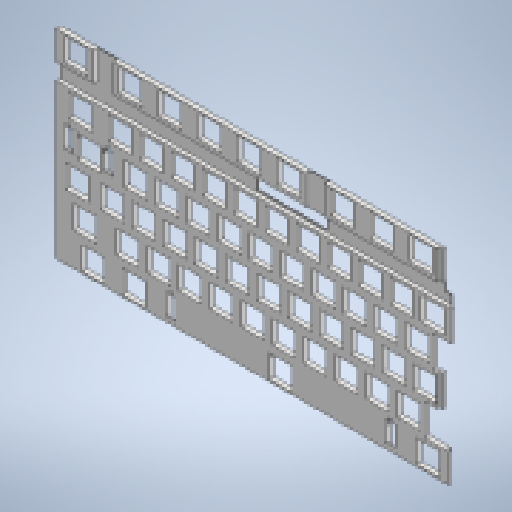
# Autodesk Inventor part: Left Plate
Saved by Autodesk Inventor 2025 (Build 290162000, 162)
## iProperties
Created: 2024-08-15
Part Number: Left Plate
Material: Generic
Document SubType Name: Modeling
Designer: adam
Density: 1 g/cm^3
Appearance: Default
Author: adam
Autodesk Inventor part; units mm, degrees
(part 1 of 2)
ref_plane "YZ Plane" through (0, 0, 0) normal (1, 0, 0) x (0, 1, 0)
ref_plane "XZ Plane" through (0, 0, 0) normal (0, 1, 0) x (-1, 0, 0)
ref_plane "XY Plane" through (0, 0, 0) normal (0, 0, 1) x (1, 0, 0)
sketch "Sketch1" plane through (0, 0, 0) normal (0, 0, 1) x (1, 0, 0)
  line L0 (356, -163) -> (40, -163) construction
  line L1 (356, -42) -> (356, -163) construction
  line L2 (40, -42) -> (356, -42) construction
  line L3 (40, -163) -> (40, -42) construction
  circle A0 centre (58.6, -159.6) radius 0.725 construction
  circle A1 centre (63, -154.9) radius 2.55 construction
  circle A2 centre (65.6, -160.65) radius 0.725 construction
  circle A3 centre (83.1, -159.6) radius 0.725 construction
  circle A4 centre (90.1, -160.65) radius 0.725 construction
  circle A5 centre (87.5, -154.9) radius 2.55 construction
  line L4 (107.125, -161.9) -> (113.125, -161.9) construction
  line L5 (107.125, -145.9) -> (107.125, -161.9) construction
  line L6 (113.125, -145.9) -> (107.125, -145.9) construction
  line L7 (113.125, -161.9) -> (113.125, -145.9) construction
  circle A6 centre (53.1, -140.5) radius 0.725 construction
  circle A7 centre (60.1, -141.55) radius 0.725 construction
  circle A8 centre (79.35, -140.5) radius 0.725 construction
  circle A9 centre (57.5, -135.8) radius 2.55 construction
  circle A10 centre (86.35, -141.55) radius 0.725 construction
  circle A11 centre (98.35, -140.5) radius 0.725 construction
  circle A12 centre (105.35, -141.55) radius 0.725 construction
  circle A13 centre (117.35, -140.5) radius 0.725 construction
  circle A14 centre (83.75, -135.8) radius 2.55 construction
  circle A15 centre (102.75, -135.8) radius 2.55 construction
  circle A16 centre (121.75, -135.8) radius 2.55 construction
  circle A17 centre (179.475, -160.65) radius 0.725 construction
  circle A18 centre (172.475, -159.6) radius 0.725 construction
  circle A19 centre (176.875, -154.9) radius 2.55 construction
  circle A20 centre (124.35, -141.55) radius 0.725 construction
  circle A21 centre (136.35, -140.5) radius 0.725 construction
  circle A22 centre (143.35, -141.55) radius 0.725 construction
  circle A23 centre (155.35, -140.5) radius 0.725 construction
  circle A24 centre (140.75, -135.8) radius 2.55 construction
  circle A25 centre (159.75, -135.8) radius 2.55 construction
  circle A26 centre (162.35, -141.55) radius 0.725 construction
  circle A27 centre (174.35, -140.5) radius 0.725 construction
  circle A28 centre (181.35, -141.55) radius 0.725 construction
  circle A29 centre (193.35, -140.5) radius 0.725 construction
  circle A30 centre (178.75, -135.8) radius 2.55 construction
  circle A31 centre (197.75, -135.8) radius 2.55 construction
  circle A32 centre (48.6, -121.4) radius 0.725 construction
  circle A33 centre (55.6, -122.45) radius 0.725 construction
  circle A34 centre (70.1, -121.4) radius 0.725 construction
  circle A35 centre (77.1, -122.45) radius 0.725 construction
  circle A36 centre (89.1, -121.4) radius 0.725 construction
  circle A37 centre (96.1, -122.45) radius 0.725 construction
  circle A38 centre (108.1, -121.4) radius 0.725 construction
  circle A39 centre (115.1, -122.45) radius 0.725 construction
  circle A40 centre (53, -116.7) radius 2.55 construction
  circle A41 centre (74.5, -116.7) radius 2.55 construction
  circle A42 centre (93.5, -116.7) radius 2.55 construction
  circle A43 centre (112.5, -116.7) radius 2.55 construction
  circle A44 centre (127.1, -121.4) radius 0.725 construction
  circle A45 centre (134.1, -122.45) radius 0.725 construction
  circle A46 centre (146.1, -121.4) radius 0.725 construction
  circle A47 centre (153.1, -122.45) radius 0.725 construction
  circle A48 centre (165.1, -121.4) radius 0.725 construction
  circle A49 centre (172.1, -122.45) radius 0.725 construction
  circle A50 centre (184.1, -121.4) radius 0.725 construction
  circle A51 centre (191.1, -122.45) radius 0.725 construction
  circle A52 centre (131.5, -116.7) radius 2.55 construction
  circle A53 centre (150.5, -116.7) radius 2.55 construction
  circle A54 centre (169.5, -116.7) radius 2.55 construction
  circle A55 centre (188.5, -116.7) radius 2.55 construction
  circle A56 centre (261.85, -159.6) radius 0.725 construction
  circle A57 centre (268.85, -160.65) radius 0.725 construction
  circle A58 centre (266.25, -154.9) radius 2.55 construction
  line L8 (240.625, -161.9) -> (246.625, -161.9) construction
  line L9 (240.625, -145.9) -> (240.625, -161.9) construction
  line L10 (246.625, -145.9) -> (240.625, -145.9) construction
  line L11 (246.625, -161.9) -> (246.625, -145.9) construction
  circle A59 centre (200.35, -141.55) radius 0.725 construction
  circle A60 centre (212.35, -140.5) radius 0.725 construction
  circle A61 centre (219.35, -141.55) radius 0.725 construction
  circle A62 centre (231.35, -140.5) radius 0.725 construction
  circle A63 centre (216.75, -135.8) radius 2.55 construction
  circle A64 centre (235.75, -135.8) radius 2.55 construction
  circle A65 centre (238.35, -141.55) radius 0.725 construction
  circle A66 centre (250.35, -140.5) radius 0.725 construction
  circle A67 centre (257.35, -141.55) radius 0.725 construction
  circle A68 centre (269.35, -140.5) radius 0.725 construction
  circle A69 centre (276.35, -141.55) radius 0.725 construction
  circle A70 centre (254.75, -135.8) radius 2.55 construction
  circle A71 centre (273.75, -135.8) radius 2.55 construction
  circle A72 centre (283.85, -159.6) radius 0.725 construction
  circle A73 centre (290.85, -160.65) radius 0.725 construction
  circle A74 centre (288.25, -154.9) radius 2.55 construction
  circle A75 centre (302.85, -159.6) radius 0.725 construction
  circle A76 centre (309.85, -160.65) radius 0.725 construction
  circle A77 centre (307.25, -154.9) radius 2.55 construction
  circle A78 centre (321.85, -159.6) radius 0.725 construction
  circle A79 centre (328.85, -160.65) radius 0.725 construction
  circle A80 centre (326.25, -154.9) radius 2.55 construction
  circle A81 centre (340.85, -159.6) radius 0.725 construction
  circle A82 centre (347.85, -160.65) radius 0.725 construction
  circle A83 centre (345.25, -154.9) radius 2.55 construction
  circle A84 centre (295.6, -140.5) radius 0.725 construction
  circle A85 centre (302.6, -141.55) radius 0.725 construction
  circle A86 centre (300, -135.8) radius 2.55 construction
  circle A87 centre (321.85, -140.5) radius 0.725 construction
  circle A88 centre (328.85, -141.55) radius 0.725 construction
  circle A89 centre (353.5, -141.62) radius 0.5 construction
  circle A90 centre (326.25, -135.8) radius 2.55 construction
  circle A91 centre (353.5, -139.08) radius 0.5 construction
  circle A92 centre (353.5, -136.54) radius 0.5 construction
  circle A93 centre (353.5, -134) radius 0.5 construction
  circle A94 centre (203.1, -121.4) radius 0.725 construction
  circle A95 centre (210.1, -122.45) radius 0.725 construction
  circle A96 centre (222.1, -121.4) radius 0.725 construction
  circle A97 centre (229.1, -122.45) radius 0.725 construction
  circle A98 centre (241.1, -121.4) radius 0.725 construction
  circle A99 centre (248.1, -122.45) radius 0.725 construction
  circle A100 centre (260.1, -121.4) radius 0.725 construction
  circle A101 centre (267.1, -122.45) radius 0.725 construction
  circle A102 centre (207.5, -116.7) radius 2.55 construction
  circle A103 centre (226.5, -116.7) radius 2.55 construction
  circle A104 centre (245.5, -116.7) radius 2.55 construction
  circle A105 centre (264.5, -116.7) radius 2.55 construction
  circle A106 centre (279.1, -121.4) radius 0.725 construction
  circle A107 centre (286.1, -122.45) radius 0.725 construction
  circle A108 centre (298.1, -121.4) radius 0.725 construction
  circle A109 centre (305.1, -122.45) radius 0.725 construction
  line L12 (315, -122.25) -> (330, -122.25) construction
  line L13 (315, -116.25) -> (315, -122.25) construction
  line L14 (330, -116.25) -> (315, -116.25) construction
  line L15 (330, -122.25) -> (330, -116.25) construction
  circle A110 centre (283.5, -116.7) radius 2.55 construction
  circle A111 centre (302.5, -116.7) radius 2.55 construction
  circle A112 centre (328.675, -111.675) radius 0.725 construction
  circle A113 centre (323.975, -107.275) radius 2.55 construction
  circle A114 centre (329.725, -104.675) radius 0.725 construction
  circle A115 centre (62.6, -103.35) radius 0.725 construction
  circle A116 centre (55.6, -102.3) radius 0.725 construction
  circle A117 centre (60, -97.6) radius 2.55 construction
  line L16 (45, -103.6) -> (51, -103.6) construction
  line L17 (45, -88.6) -> (45, -103.6) construction
  line L18 (51, -88.6) -> (45, -88.6) construction
  line L19 (51, -103.6) -> (51, -88.6) construction
  line L20 (69, -103.6) -> (75, -103.6) construction
  line L21 (69, -88.6) -> (69, -103.6) construction
  line L22 (75, -88.6) -> (69, -88.6) construction
  line L23 (75, -103.6) -> (75, -88.6) construction
  circle A118 centre (91.35, -103.35) radius 0.725 construction
  circle A119 centre (84.35, -102.3) radius 0.725 construction
  circle A120 centre (88.75, -97.6) radius 2.55 construction
  circle A121 centre (110.35, -103.35) radius 0.725 construction
  circle A122 centre (103.35, -102.3) radius 0.725 construction
  circle A123 centre (107.75, -97.6) radius 2.55 construction
  circle A124 centre (57.6, -84.25) radius 0.725 construction
  circle A125 centre (81.6, -84.25) radius 0.725 construction
  circle A126 centre (50.6, -83.2) radius 0.725 construction
  circle A127 centre (55, -78.5) radius 2.55 construction
  circle A128 centre (74.6, -83.2) radius 0.725 construction
  circle A129 centre (79, -78.5) radius 2.55 construction
  circle A130 centre (100.6, -84.25) radius 0.725 construction
  circle A131 centre (119.6, -84.25) radius 0.725 construction
  circle A132 centre (93.6, -83.2) radius 0.725 construction
  circle A133 centre (98, -78.5) radius 2.55 construction
  circle A134 centre (112.6, -83.2) radius 0.725 construction
  circle A135 centre (117, -78.5) radius 2.55 construction
  circle A136 centre (129.35, -103.35) radius 0.725 construction
  circle A137 centre (122.35, -102.3) radius 0.725 construction
  circle A138 centre (141.35, -102.3) radius 0.725 construction
  circle A139 centre (126.75, -97.6) radius 2.55 construction
  circle A140 centre (148.35, -103.35) radius 0.725 construction
  circle A141 centre (160.35, -102.3) radius 0.725 construction
  circle A142 centre (145.75, -97.6) radius 2.55 construction
  circle A143 centre (167.35, -103.35) radius 0.725 construction
  circle A144 centre (179.35, -102.3) radius 0.725 construction
  circle A145 centre (164.75, -97.6) radius 2.55 construction
  circle A146 centre (186.35, -103.35) radius 0.725 construction
  circle A147 centre (198.35, -102.3) radius 0.725 construction
  circle A148 centre (183.75, -97.6) radius 2.55 construction
  circle A149 centre (138.6, -84.25) radius 0.725 construction
  circle A150 centre (157.6, -84.25) radius 0.725 construction
  circle A151 centre (131.6, -83.2) radius 0.725 construction
  circle A152 centre (136, -78.5) radius 2.55 construction
  circle A153 centre (150.6, -83.2) radius 0.725 construction
  circle A154 centre (155, -78.5) radius 2.55 construction
  circle A155 centre (176.6, -84.25) radius 0.725 construction
  circle A156 centre (195.6, -84.25) radius 0.725 construction
  circle A157 centre (169.6, -83.2) radius 0.725 construction
  circle A158 centre (174, -78.5) radius 2.55 construction
  circle A159 centre (188.6, -83.2) radius 0.725 construction
  circle A160 centre (193, -78.5) radius 2.55 construction
  circle A161 centre (48.1, -54.7) radius 0.725 construction
  circle A162 centre (55.1, -55.75) radius 0.725 construction
  circle A163 centre (81.1, -54.7) radius 0.725 construction
  circle A164 centre (52.5, -50) radius 2.55 construction
  circle A165 centre (88.1, -55.75) radius 0.725 construction
  circle A166 centre (105.1, -54.7) radius 0.725 construction
  circle A167 centre (112.1, -55.75) radius 0.725 construction
  circle A168 centre (85.5, -50) radius 2.55 construction
  circle A169 centre (109.5, -50) radius 2.55 construction
  circle A170 centre (163.5, -66.25) radius 0.425 construction
  circle A171 centre (166, -66.25) radius 0.425 construction
  circle A172 centre (168.5, -66.25) radius 0.425 construction
  circle A173 centre (171, -66.25) radius 0.425 construction
  circle A174 centre (173.5, -66.25) radius 0.425 construction
  circle A175 centre (176, -66.25) radius 0.425 construction
  circle A176 centre (178.5, -66.25) radius 0.425 construction
  circle A177 centre (162.25, -63.75) radius 0.425 construction
  circle A178 centre (164.75, -63.75) radius 0.425 construction
  circle A179 centre (167.25, -63.75) radius 0.425 construction
  circle A180 centre (169.75, -63.75) radius 0.425 construction
  circle A181 centre (172.25, -63.75) radius 0.425 construction
  circle A182 centre (174.75, -63.75) radius 0.425 construction
  circle A183 centre (177.25, -63.75) radius 0.425 construction
  circle A184 centre (179.75, -63.75) radius 0.425 construction
  circle A185 centre (181, -66.25) radius 0.425 construction
  circle A186 centre (183.5, -66.25) radius 0.425 construction
  circle A187 centre (186, -66.25) radius 0.425 construction
  circle A188 centre (188.5, -66.25) radius 0.425 construction
  circle A189 centre (191, -66.25) radius 0.425 construction
  circle A190 centre (193.5, -66.25) radius 0.425 construction
  circle A191 centre (196, -66.25) radius 0.425 construction
  circle A192 centre (198.5, -66.25) radius 0.425 construction
  circle A193 centre (182.25, -63.75) radius 0.425 construction
  circle A194 centre (184.75, -63.75) radius 0.425 construction
  circle A195 centre (187.25, -63.75) radius 0.425 construction
  circle A196 centre (189.75, -63.75) radius 0.425 construction
  circle A197 centre (192.25, -63.75) radius 0.425 construction
  circle A198 centre (194.75, -63.75) radius 0.425 construction
  circle A199 centre (197.25, -63.75) radius 0.425 construction
  circle A200 centre (129.1, -54.7) radius 0.725 construction
  circle A201 centre (136.1, -55.75) radius 0.725 construction
  circle A202 centre (153.1, -54.7) radius 0.725 construction
  circle A203 centre (160.1, -55.75) radius 0.725 construction
  circle A204 centre (133.5, -50) radius 2.55 construction
  circle A205 centre (157.5, -50) radius 2.55 construction
  circle A206 centre (177.1, -54.7) radius 0.725 construction
  circle A207 centre (184.1, -55.75) radius 0.725 construction
  circle A208 centre (181.5, -50) radius 2.55 construction
  circle A209 centre (205.35, -103.35) radius 0.725 construction
  circle A210 centre (217.35, -102.3) radius 0.725 construction
  circle A211 centre (202.75, -97.6) radius 2.55 construction
  circle A212 centre (224.35, -103.35) radius 0.725 construction
  circle A213 centre (236.35, -102.3) radius 0.725 construction
  circle A214 centre (221.75, -97.6) radius 2.55 construction
  circle A215 centre (243.35, -103.35) radius 0.725 construction
  circle A216 centre (255.35, -102.3) radius 0.725 construction
  circle A217 centre (240.75, -97.6) radius 2.55 construction
  circle A218 centre (262.35, -103.35) radius 0.725 construction
  circle A219 centre (274.35, -102.3) radius 0.725 construction
  circle A220 centre (259.75, -97.6) radius 2.55 construction
  circle A221 centre (214.6, -84.25) radius 0.725 construction
  circle A222 centre (233.6, -84.25) radius 0.725 construction
  circle A223 centre (207.6, -83.2) radius 0.725 construction
  circle A224 centre (212, -78.5) radius 2.55 construction
  circle A225 centre (226.6, -83.2) radius 0.725 construction
  circle A226 centre (231, -78.5) radius 2.55 construction
  circle A227 centre (252.6, -84.25) radius 0.725 construction
  circle A228 centre (271.6, -84.25) radius 0.725 construction
  circle A229 centre (245.6, -83.2) radius 0.725 construction
  circle A230 centre (250, -78.5) radius 2.55 construction
  circle A231 centre (264.6, -83.2) radius 0.725 construction
  circle A232 centre (269, -78.5) radius 2.55 construction
  circle A233 centre (281.35, -103.35) radius 0.725 construction
  circle A234 centre (293.35, -102.3) radius 0.725 construction
  circle A235 centre (278.75, -97.6) radius 2.55 construction
  circle A236 centre (300.35, -103.35) radius 0.725 construction
  circle A237 centre (297.75, -97.6) radius 2.55 construction
  line L24 (315, -98.25) -> (330, -98.25) construction
  line L25 (315, -92.25) -> (315, -98.25) construction
  line L26 (330, -92.25) -> (315, -92.25) construction
  line L27 (330, -98.25) -> (330, -92.25) construction
  circle A238 centre (290.6, -84.25) radius 0.725 construction
  circle A239 centre (309.6, -84.25) radius 0.725 construction
  circle A240 centre (283.6, -83.2) radius 0.725 construction
  circle A241 centre (288, -78.5) radius 2.55 construction
  circle A242 centre (302.6, -83.2) radius 0.725 construction
  circle A243 centre (307, -78.5) radius 2.55 construction
  circle A244 centre (328.6, -84.25) radius 0.725 construction
  circle A245 centre (347.6, -84.25) radius 0.725 construction
  circle A246 centre (321.6, -83.2) radius 0.725 construction
  circle A247 centre (326, -78.5) radius 2.55 construction
  circle A248 centre (340.6, -83.2) radius 0.725 construction
  circle A249 centre (345, -78.5) radius 2.55 construction
  circle A250 centre (201, -66.25) radius 0.425 construction
  circle A251 centre (199.75, -63.75) radius 0.425 construction
  circle A252 centre (259, -74) radius 1.6 construction
  circle A253 centre (209.6, -54.7) radius 0.725 construction
  circle A254 centre (216.6, -55.75) radius 0.725 construction
  circle A255 centre (233.6, -54.7) radius 0.725 construction
  circle A256 centre (214, -50) radius 2.55 construction
  circle A257 centre (238, -50) radius 2.55 construction
  circle A258 centre (240.6, -55.75) radius 0.725 construction
  circle A259 centre (257.6, -54.7) radius 0.725 construction
  circle A260 centre (264.6, -55.75) radius 0.725 construction
  circle A261 centre (262, -50) radius 2.55 construction
  circle A262 centre (281.6, -54.7) radius 0.725 construction
  circle A263 centre (288.6, -55.75) radius 0.725 construction
  circle A264 centre (305.6, -54.7) radius 0.725 construction
  circle A265 centre (312.6, -55.75) radius 0.725 construction
  circle A266 centre (286, -50) radius 2.55 construction
  circle A267 centre (310, -50) radius 2.55 construction
  circle A268 centre (339.1, -54.7) radius 0.725 construction
  circle A269 centre (346.1, -55.75) radius 0.725 construction
  circle A270 centre (343.5, -50) radius 2.55 construction
  line L28 (277.25, -163) -> (277.25, -145.35) construction
  line L29 (277.25, -145.35) -> (264.25, -145.35) construction
  line L30 (264.25, -145.35) -> (264.25, -126.25) construction
  line L31 (264.25, -126.25) -> (274, -126.25) construction
  line L32 (274, -126.25) -> (274, -107.15) construction
  line L33 (274, -107.15) -> (269.25, -107.15) construction
  line L34 (269.25, -107.15) -> (269.25, -88.05) construction
  line L35 (269.25, -88.05) -> (278.5, -88.05) construction
  line L36 (278.5, -88.05) -> (278.5, -64.25) construction
  line L37 (274, -42) -> (274, -64.25) construction
  line L38 (274, -64.25) -> (278.5, -64.25) construction
  line L39 (262, -50) -> (274, -50) construction
  line L40 (274, -50) -> (286, -50) construction
  line L41 (269, -78.5) -> (278.5, -78.5) construction
  line L42 (278.5, -78.5) -> (288, -78.5) construction
  line L43 (259.75, -97.6) -> (269.25, -97.6) construction
  line L44 (269.25, -97.6) -> (278.75, -97.6) construction
  line L45 (264.5, -116.7) -> (274, -116.7) construction
  line L46 (283.5, -116.7) -> (274, -116.7) construction
  line L47 (254.75, -135.8) -> (264.25, -135.8) construction
  line L48 (273.75, -135.8) -> (264.25, -135.8) construction
  line L49 (266.25, -154.9) -> (277.25, -154.9) construction
  line L50 (288.25, -154.9) -> (277.25, -154.9) construction
  line L51 (273.75, -135.8) -> (273.75, -145.35) construction
  line L52 (273.75, -145.35) -> (273.75, -154.9) construction
  line L53 (269.35, -140.5) -> (269.35, -135.8) construction
  line L54 (269.35, -135.8) -> (269.35, -126.25) construction
  line L55 (269.35, -126.25) -> (269.35, -116.7) construction
  line L56 (271.75, -116.7) -> (271.75, -107.15) construction
  line L57 (271.75, -107.15) -> (271.75, -97.6) construction
  line L58 (271.75, -97.6) -> (271.75, -88.05) construction
  line L59 (271.75, -88.05) -> (271.75, -78.5) construction
  line L60 (276.25, -78.5) -> (276.25, -64.25) construction
  line L61 (276.25, -64.25) -> (276.25, -50) construction
  line L62 (273.9, -126.15) -> (264.15, -126.15)
  line L63 (264.15, -126.15) -> (264.15, -145.45)
  line L64 (264.15, -145.45) -> (277.15, -145.45)
  line L65 (277.15, -145.45) -> (277.15, -163)
  line L66 (277.15, -163) -> (40, -163)
  line L67 (40, -163) -> (40, -42)
  line L68 (40, -42) -> (273.9, -42)
  line L69 (273.9, -126.15) -> (273.9, -107.25)
  line L70 (273.9, -107.25) -> (269.15, -107.25)
  line L71 (269.15, -107.25) -> (269.15, -87.95)
  line L72 (269.15, -87.95) -> (278.4, -87.95)
  line L73 (278.4, -87.95) -> (278.4, -64.35)
  line L74 (278.4, -64.35) -> (273.9, -64.35)
  line L75 (273.9, -64.35) -> (273.9, -42)
  line L76 (45.4975, -42.9975) -> (59.5025, -42.9975)
  line L77 (59.5025, -42.9975) -> (59.5025, -57.0025)
  line L78 (59.5025, -57.0025) -> (45.4975, -57.0025)
  line L79 (45.4975, -57.0025) -> (45.4975, -42.9975)
  line L80 (45.4975, -42.9975) -> (59.5025, -57.0025) construction
  line L81 (59.5025, -42.9975) -> (45.4975, -57.0025) construction
  line L82 (78.4975, -42.9975) -> (92.5025, -42.9975)
  line L83 (92.5025, -42.9975) -> (92.5025, -57.0025)
  line L84 (92.5025, -57.0025) -> (78.4975, -57.0025)
  line L85 (78.4975, -57.0025) -> (78.4975, -42.9975)
  line L86 (78.4975, -42.9975) -> (92.5025, -57.0025) construction
  line L87 (92.5025, -42.9975) -> (78.4975, -57.0025) construction
  line L88 (102.4975, -42.9975) -> (116.5025, -42.9975)
  line L89 (116.5025, -42.9975) -> (116.5025, -57.0025)
  line L90 (116.5025, -57.0025) -> (102.4975, -57.0025)
  line L91 (102.4975, -57.0025) -> (102.4975, -42.9975)
  line L92 (102.4975, -42.9975) -> (116.5025, -57.0025) construction
  line L93 (116.5025, -42.9975) -> (102.4975, -57.0025) construction
  line L94 (126.4975, -42.9975) -> (140.5025, -42.9975)
  line L95 (140.5025, -42.9975) -> (140.5025, -57.0025)
  line L96 (140.5025, -57.0025) -> (126.4975, -57.0025)
  line L97 (126.4975, -57.0025) -> (126.4975, -42.9975)
  line L98 (126.4975, -42.9975) -> (140.5025, -57.0025) construction
  line L99 (140.5025, -42.9975) -> (126.4975, -57.0025) construction
  line L100 (150.4975, -42.9975) -> (164.5025, -42.9975)
  line L101 (164.5025, -42.9975) -> (164.5025, -57.0025)
  line L102 (164.5025, -57.0025) -> (150.4975, -57.0025)
  line L103 (150.4975, -57.0025) -> (150.4975, -42.9975)
  line L104 (150.4975, -42.9975) -> (164.5025, -57.0025) construction
  line L105 (164.5025, -42.9975) -> (150.4975, -57.0025) construction
  line L106 (174.4975, -42.9975) -> (188.5025, -42.9975)
  line L107 (188.5025, -42.9975) -> (188.5025, -57.0025)
  line L108 (188.5025, -57.0025) -> (174.4975, -57.0025)
  line L109 (174.4975, -57.0025) -> (174.4975, -42.9975)
  line L110 (174.4975, -42.9975) -> (188.5025, -57.0025) construction
  line L111 (188.5025, -42.9975) -> (174.4975, -57.0025) construction
  line L112 (206.9975, -42.9975) -> (221.0025, -42.9975)
  line L113 (221.0025, -42.9975) -> (221.0025, -57.0025)
  line L114 (221.0025, -57.0025) -> (206.9975, -57.0025)
  line L115 (206.9975, -57.0025) -> (206.9975, -42.9975)
  line L116 (206.9975, -42.9975) -> (221.0025, -57.0025) construction
  line L117 (221.0025, -42.9975) -> (206.9975, -57.0025) construction
  line L118 (230.9975, -42.9975) -> (245.0025, -42.9975)
  line L119 (245.0025, -42.9975) -> (245.0025, -57.0025)
  line L120 (245.0025, -57.0025) -> (230.9975, -57.0025)
  line L121 (230.9975, -57.0025) -> (230.9975, -42.9975)
  line L122 (230.9975, -42.9975) -> (245.0025, -57.0025) construction
  line L123 (245.0025, -42.9975) -> (230.9975, -57.0025) construction
  line L124 (254.9975, -42.9975) -> (269.0025, -42.9975)
  line L125 (269.0025, -42.9975) -> (269.0025, -57.0025)
  line L126 (269.0025, -57.0025) -> (254.9975, -57.0025)
  line L127 (254.9975, -57.0025) -> (254.9975, -42.9975)
  line L128 (254.9975, -42.9975) -> (269.0025, -57.0025) construction
  line L129 (269.0025, -42.9975) -> (254.9975, -57.0025) construction
  line L130 (47.9975, -71.4975) -> (62.0025, -71.4975)
  line L131 (62.0025, -71.4975) -> (62.0025, -85.5025)
  line L132 (62.0025, -85.5025) -> (47.9975, -85.5025)
  line L133 (47.9975, -85.5025) -> (47.9975, -71.4975)
  line L134 (47.9975, -71.4975) -> (62.0025, -85.5025) construction
  line L135 (62.0025, -71.4975) -> (47.9975, -85.5025) construction
  line L136 (71.9975, -71.4975) -> (86.0025, -71.4975)
  line L137 (86.0025, -71.4975) -> (86.0025, -85.5025)
  line L138 (86.0025, -85.5025) -> (71.9975, -85.5025)
  line L139 (71.9975, -85.5025) -> (71.9975, -71.4975)
  line L140 (71.9975, -71.4975) -> (86.0025, -85.5025) construction
  line L141 (86.0025, -71.4975) -> (71.9975, -85.5025) construction
  line L142 (90.9975, -71.4975) -> (105.0025, -71.4975)
  line L143 (105.0025, -71.4975) -> (105.0025, -85.5025)
  line L144 (105.0025, -85.5025) -> (90.9975, -85.5025)
  line L145 (90.9975, -85.5025) -> (90.9975, -71.4975)
  line L146 (90.9975, -71.4975) -> (105.0025, -85.5025) construction
  line L147 (105.0025, -71.4975) -> (90.9975, -85.5025) construction
  line L148 (109.9975, -71.4975) -> (124.0025, -71.4975)
  line L149 (124.0025, -71.4975) -> (124.0025, -85.5025)
  line L150 (124.0025, -85.5025) -> (109.9975, -85.5025)
  line L151 (109.9975, -85.5025) -> (109.9975, -71.4975)
  line L152 (109.9975, -71.4975) -> (124.0025, -85.5025) construction
  line L153 (124.0025, -71.4975) -> (109.9975, -85.5025) construction
  line L154 (128.9975, -71.4975) -> (143.0025, -71.4975)
  line L155 (143.0025, -71.4975) -> (143.0025, -85.5025)
  line L156 (143.0025, -85.5025) -> (128.9975, -85.5025)
  line L157 (128.9975, -85.5025) -> (128.9975, -71.4975)
  line L158 (128.9975, -71.4975) -> (143.0025, -85.5025) construction
  line L159 (143.0025, -71.4975) -> (128.9975, -85.5025) construction
  line L160 (147.9975, -71.4975) -> (162.0025, -71.4975)
  line L161 (162.0025, -71.4975) -> (162.0025, -85.5025)
  line L162 (162.0025, -85.5025) -> (147.9975, -85.5025)
  line L163 (147.9975, -85.5025) -> (147.9975, -71.4975)
  line L164 (147.9975, -71.4975) -> (162.0025, -85.5025) construction
  line L165 (162.0025, -71.4975) -> (147.9975, -85.5025) construction
  line L166 (166.9975, -71.4975) -> (181.0025, -71.4975)
  line L167 (181.0025, -71.4975) -> (181.0025, -85.5025)
  line L168 (181.0025, -85.5025) -> (166.9975, -85.5025)
  line L169 (166.9975, -85.5025) -> (166.9975, -71.4975)
  line L170 (166.9975, -71.4975) -> (181.0025, -85.5025) construction
  line L171 (181.0025, -71.4975) -> (166.9975, -85.5025) construction
  line L172 (185.9975, -71.4975) -> (200.0025, -71.4975)
  line L173 (200.0025, -71.4975) -> (200.0025, -85.5025)
  line L174 (200.0025, -85.5025) -> (185.9975, -85.5025)
  line L175 (185.9975, -85.5025) -> (185.9975, -71.4975)
  line L176 (185.9975, -71.4975) -> (200.0025, -85.5025) construction
  line L177 (200.0025, -71.4975) -> (185.9975, -85.5025) construction
  line L178 (204.9975, -71.4975) -> (219.0025, -71.4975)
  line L179 (219.0025, -71.4975) -> (219.0025, -85.5025)
  line L180 (219.0025, -85.5025) -> (204.9975, -85.5025)
  line L181 (204.9975, -85.5025) -> (204.9975, -71.4975)
  line L182 (204.9975, -71.4975) -> (219.0025, -85.5025) construction
  line L183 (219.0025, -71.4975) -> (204.9975, -85.5025) construction
  line L184 (223.9975, -71.4975) -> (238.0025, -71.4975)
  line L185 (238.0025, -71.4975) -> (238.0025, -85.5025)
  line L186 (238.0025, -85.5025) -> (223.9975, -85.5025)
  line L187 (223.9975, -85.5025) -> (223.9975, -71.4975)
  line L188 (223.9975, -71.4975) -> (238.0025, -85.5025) construction
  line L189 (238.0025, -71.4975) -> (223.9975, -85.5025) construction
  line L190 (242.9975, -71.4975) -> (257.0025, -71.4975)
  line L191 (257.0025, -71.4975) -> (257.0025, -85.5025)
  line L192 (257.0025, -85.5025) -> (242.9975, -85.5025)
  line L193 (242.9975, -85.5025) -> (242.9975, -71.4975)
  line L194 (242.9975, -71.4975) -> (257.0025, -85.5025) construction
  line L195 (257.0025, -71.4975) -> (242.9975, -85.5025) construction
  line L196 (261.9975, -71.4975) -> (276.0025, -71.4975)
  line L197 (276.0025, -71.4975) -> (276.0025, -85.5025)
  line L198 (276.0025, -85.5025) -> (261.9975, -85.5025)
  line L199 (261.9975, -85.5025) -> (261.9975, -71.4975)
  line L200 (261.9975, -71.4975) -> (276.0025, -85.5025) construction
  line L201 (276.0025, -71.4975) -> (261.9975, -85.5025) construction
  line L202 (52.9975, -90.5975) -> (67.0025, -90.5975)
  line L203 (67.0025, -90.5975) -> (67.0025, -104.6025)
  line L204 (67.0025, -104.6025) -> (52.9975, -104.6025)
  line L205 (52.9975, -104.6025) -> (52.9975, -90.5975)
  line L206 (52.9975, -90.5975) -> (67.0025, -104.6025) construction
  line L207 (67.0025, -90.5975) -> (52.9975, -104.6025) construction
  line L208 (81.7475, -90.5975) -> (95.7525, -90.5975)
  line L209 (95.7525, -90.5975) -> (95.7525, -104.6025)
  line L210 (95.7525, -104.6025) -> (81.7475, -104.6025)
  line L211 (81.7475, -104.6025) -> (81.7475, -90.5975)
  line L212 (81.7475, -90.5975) -> (95.7525, -104.6025) construction
  line L213 (95.7525, -90.5975) -> (81.7475, -104.6025) construction
  line L214 (100.7475, -90.5975) -> (114.7525, -90.5975)
  line L215 (114.7525, -90.5975) -> (114.7525, -104.6025)
  line L216 (114.7525, -104.6025) -> (100.7475, -104.6025)
  line L217 (100.7475, -104.6025) -> (100.7475, -90.5975)
  line L218 (100.7475, -90.5975) -> (114.7525, -104.6025) construction
  line L219 (114.7525, -90.5975) -> (100.7475, -104.6025) construction
  line L220 (119.7475, -90.5975) -> (133.7525, -90.5975)
  line L221 (133.7525, -90.5975) -> (133.7525, -104.6025)
  line L222 (133.7525, -104.6025) -> (119.7475, -104.6025)
  line L223 (119.7475, -104.6025) -> (119.7475, -90.5975)
  line L224 (119.7475, -90.5975) -> (133.7525, -104.6025) construction
  line L225 (133.7525, -90.5975) -> (119.7475, -104.6025) construction
  line L226 (138.7475, -90.5975) -> (152.7525, -90.5975)
  line L227 (152.7525, -90.5975) -> (152.7525, -104.6025)
  line L228 (152.7525, -104.6025) -> (138.7475, -104.6025)
  line L229 (138.7475, -104.6025) -> (138.7475, -90.5975)
  line L230 (138.7475, -90.5975) -> (152.7525, -104.6025) construction
  line L231 (152.7525, -90.5975) -> (138.7475, -104.6025) construction
  line L232 (157.7475, -90.5975) -> (171.7525, -90.5975)
  line L233 (171.7525, -90.5975) -> (171.7525, -104.6025)
  line L234 (171.7525, -104.6025) -> (157.7475, -104.6025)
  line L235 (157.7475, -104.6025) -> (157.7475, -90.5975)
  line L236 (157.7475, -90.5975) -> (171.7525, -104.6025) construction
  line L237 (171.7525, -90.5975) -> (157.7475, -104.6025) construction
  line L238 (176.7475, -90.5975) -> (190.7525, -90.5975)
  line L239 (190.7525, -90.5975) -> (190.7525, -104.6025)
  line L240 (190.7525, -104.6025) -> (176.7475, -104.6025)
  line L241 (176.7475, -104.6025) -> (176.7475, -90.5975)
  line L242 (176.7475, -90.5975) -> (190.7525, -104.6025) construction
  line L243 (190.7525, -90.5975) -> (176.7475, -104.6025) construction
  line L244 (195.7475, -90.5975) -> (209.7525, -90.5975)
  line L245 (209.7525, -90.5975) -> (209.7525, -104.6025)
  line L246 (209.7525, -104.6025) -> (195.7475, -104.6025)
  line L247 (195.7475, -104.6025) -> (195.7475, -90.5975)
  line L248 (195.7475, -90.5975) -> (209.7525, -104.6025) construction
  line L249 (209.7525, -90.5975) -> (195.7475, -104.6025) construction
  line L250 (214.7475, -90.5975) -> (228.7525, -90.5975)
  line L251 (228.7525, -90.5975) -> (228.7525, -104.6025)
  line L252 (228.7525, -104.6025) -> (214.7475, -104.6025)
  line L253 (214.7475, -104.6025) -> (214.7475, -90.5975)
  line L254 (214.7475, -90.5975) -> (228.7525, -104.6025) construction
  line L255 (228.7525, -90.5975) -> (214.7475, -104.6025) construction
  line L256 (233.7475, -90.5975) -> (247.7525, -90.5975)
  line L257 (247.7525, -90.5975) -> (247.7525, -104.6025)
  line L258 (247.7525, -104.6025) -> (233.7475, -104.6025)
  line L259 (233.7475, -104.6025) -> (233.7475, -90.5975)
  line L260 (233.7475, -90.5975) -> (247.7525, -104.6025) construction
  line L261 (247.7525, -90.5975) -> (233.7475, -104.6025) construction
  line L262 (252.7475, -90.5975) -> (266.7525, -90.5975)
  line L263 (266.7525, -90.5975) -> (266.7525, -104.6025)
  line L264 (266.7525, -104.6025) -> (252.7475, -104.6025)
  line L265 (252.7475, -104.6025) -> (252.7475, -90.5975)
  line L266 (252.7475, -90.5975) -> (266.7525, -104.6025) construction
  line L267 (266.7525, -90.5975) -> (252.7475, -104.6025) construction
  line L268 (45.9975, -109.6975) -> (60.0025, -109.6975)
  line L269 (60.0025, -109.6975) -> (60.0025, -123.7025)
  line L270 (60.0025, -123.7025) -> (45.9975, -123.7025)
  line L271 (45.9975, -123.7025) -> (45.9975, -109.6975)
  line L272 (45.9975, -109.6975) -> (60.0025, -123.7025) construction
  line L273 (60.0025, -109.6975) -> (45.9975, -123.7025) construction
  line L274 (67.4975, -109.6975) -> (81.5025, -109.6975)
  line L275 (81.5025, -109.6975) -> (81.5025, -123.7025)
  line L276 (81.5025, -123.7025) -> (67.4975, -123.7025)
  line L277 (67.4975, -123.7025) -> (67.4975, -109.6975)
  line L278 (67.4975, -109.6975) -> (81.5025, -123.7025) construction
  line L279 (81.5025, -109.6975) -> (67.4975, -123.7025) construction
  line L280 (86.4975, -109.6975) -> (100.5025, -109.6975)
  line L281 (100.5025, -109.6975) -> (100.5025, -123.7025)
  line L282 (100.5025, -123.7025) -> (86.4975, -123.7025)
  line L283 (86.4975, -123.7025) -> (86.4975, -109.6975)
  line L284 (86.4975, -109.6975) -> (100.5025, -123.7025) construction
  line L285 (100.5025, -109.6975) -> (86.4975, -123.7025) construction
  line L286 (105.4975, -109.6975) -> (119.5025, -109.6975)
  line L287 (119.5025, -109.6975) -> (119.5025, -123.7025)
  line L288 (119.5025, -123.7025) -> (105.4975, -123.7025)
  line L289 (105.4975, -123.7025) -> (105.4975, -109.6975)
  line L290 (105.4975, -109.6975) -> (119.5025, -123.7025) construction
  line L291 (119.5025, -109.6975) -> (105.4975, -123.7025) construction
  line L292 (124.4975, -109.6975) -> (138.5025, -109.6975)
  line L293 (138.5025, -109.6975) -> (138.5025, -123.7025)
  line L294 (138.5025, -123.7025) -> (124.4975, -123.7025)
  line L295 (124.4975, -123.7025) -> (124.4975, -109.6975)
  line L296 (124.4975, -109.6975) -> (138.5025, -123.7025) construction
  line L297 (138.5025, -109.6975) -> (124.4975, -123.7025) construction
  line L298 (143.4975, -109.6975) -> (157.5025, -109.6975)
  line L299 (157.5025, -109.6975) -> (157.5025, -123.7025)
  line L300 (157.5025, -123.7025) -> (143.4975, -123.7025)
  line L301 (143.4975, -123.7025) -> (143.4975, -109.6975)
  line L302 (143.4975, -109.6975) -> (157.5025, -123.7025) construction
  line L303 (157.5025, -109.6975) -> (143.4975, -123.7025) construction
  line L304 (162.4975, -109.6975) -> (176.5025, -109.6975)
  line L305 (176.5025, -109.6975) -> (176.5025, -123.7025)
  line L306 (176.5025, -123.7025) -> (162.4975, -123.7025)
  line L307 (162.4975, -123.7025) -> (162.4975, -109.6975)
  line L308 (162.4975, -109.6975) -> (176.5025, -123.7025) construction
  line L309 (176.5025, -109.6975) -> (162.4975, -123.7025) construction
  line L310 (181.4975, -109.6975) -> (195.5025, -109.6975)
  line L311 (195.5025, -109.6975) -> (195.5025, -123.7025)
  line L312 (195.5025, -123.7025) -> (181.4975, -123.7025)
  line L313 (181.4975, -123.7025) -> (181.4975, -109.6975)
  line L314 (181.4975, -109.6975) -> (195.5025, -123.7025) construction
  line L315 (195.5025, -109.6975) -> (181.4975, -123.7025) construction
  line L316 (200.4975, -109.6975) -> (214.5025, -109.6975)
  line L317 (214.5025, -109.6975) -> (214.5025, -123.7025)
  line L318 (214.5025, -123.7025) -> (200.4975, -123.7025)
  line L319 (200.4975, -123.7025) -> (200.4975, -109.6975)
  line L320 (200.4975, -109.6975) -> (214.5025, -123.7025) construction
  line L321 (214.5025, -109.6975) -> (200.4975, -123.7025) construction
  line L322 (219.4975, -109.6975) -> (233.5025, -109.6975)
  line L323 (233.5025, -109.6975) -> (233.5025, -123.7025)
  line L324 (233.5025, -123.7025) -> (219.4975, -123.7025)
  line L325 (219.4975, -123.7025) -> (219.4975, -109.6975)
  line L326 (219.4975, -109.6975) -> (233.5025, -123.7025) construction
  line L327 (233.5025, -109.6975) -> (219.4975, -123.7025) construction
  line L328 (238.4975, -109.6975) -> (252.5025, -109.6975)
  line L329 (252.5025, -109.6975) -> (252.5025, -123.7025)
  line L330 (252.5025, -123.7025) -> (238.4975, -123.7025)
  line L331 (238.4975, -123.7025) -> (238.4975, -109.6975)
  line L332 (238.4975, -109.6975) -> (252.5025, -123.7025) construction
  line L333 (252.5025, -109.6975) -> (238.4975, -123.7025) construction
  line L334 (257.4975, -109.6975) -> (271.5025, -109.6975)
  line L335 (271.5025, -109.6975) -> (271.5025, -123.7025)
  line L336 (271.5025, -123.7025) -> (257.4975, -123.7025)
  line L337 (257.4975, -123.7025) -> (257.4975, -109.6975)
  line L338 (257.4975, -109.6975) -> (271.5025, -123.7025) construction
  line L339 (271.5025, -109.6975) -> (257.4975, -123.7025) construction
  line L340 (50.4975, -128.7975) -> (64.5025, -128.7975)
  line L341 (64.5025, -128.7975) -> (64.5025, -142.8025)
  line L342 (64.5025, -142.8025) -> (50.4975, -142.8025)
  line L343 (50.4975, -142.8025) -> (50.4975, -128.7975)
  line L344 (50.4975, -128.7975) -> (64.5025, -142.8025) construction
  line L345 (64.5025, -128.7975) -> (50.4975, -142.8025) construction
  line L346 (76.7475, -128.7975) -> (90.7525, -128.7975)
  line L347 (90.7525, -128.7975) -> (90.7525, -142.8025)
  line L348 (90.7525, -142.8025) -> (76.7475, -142.8025)
  line L349 (76.7475, -142.8025) -> (76.7475, -128.7975)
  line L350 (76.7475, -128.7975) -> (90.7525, -142.8025) construction
  line L351 (90.7525, -128.7975) -> (76.7475, -142.8025) construction
  line L352 (95.7475, -128.7975) -> (109.7525, -128.7975)
  line L353 (109.7525, -128.7975) -> (109.7525, -142.8025)
  line L354 (109.7525, -142.8025) -> (95.7475, -142.8025)
  line L355 (95.7475, -142.8025) -> (95.7475, -128.7975)
  line L356 (95.7475, -128.7975) -> (109.7525, -142.8025) construction
  line L357 (109.7525, -128.7975) -> (95.7475, -142.8025) construction
  line L358 (114.7475, -128.7975) -> (128.7525, -128.7975)
  line L359 (128.7525, -128.7975) -> (128.7525, -142.8025)
  line L360 (128.7525, -142.8025) -> (114.7475, -142.8025)
  line L361 (114.7475, -142.8025) -> (114.7475, -128.7975)
  line L362 (114.7475, -128.7975) -> (128.7525, -142.8025) construction
  line L363 (128.7525, -128.7975) -> (114.7475, -142.8025) construction
  line L364 (133.7475, -128.7975) -> (147.7525, -128.7975)
  line L365 (147.7525, -128.7975) -> (147.7525, -142.8025)
  line L366 (147.7525, -142.8025) -> (133.7475, -142.8025)
  line L367 (133.7475, -142.8025) -> (133.7475, -128.7975)
  line L368 (133.7475, -128.7975) -> (147.7525, -142.8025) construction
  line L369 (147.7525, -128.7975) -> (133.7475, -142.8025) construction
  line L370 (152.7475, -128.7975) -> (166.7525, -128.7975)
  line L371 (166.7525, -128.7975) -> (166.7525, -142.8025)
  line L372 (166.7525, -142.8025) -> (152.7475, -142.8025)
  line L373 (152.7475, -142.8025) -> (152.7475, -128.7975)
  line L374 (152.7475, -128.7975) -> (166.7525, -142.8025) construction
  line L375 (166.7525, -128.7975) -> (152.7475, -142.8025) construction
  line L376 (171.7475, -128.7975) -> (185.7525, -128.7975)
  line L377 (185.7525, -128.7975) -> (185.7525, -142.8025)
  line L378 (185.7525, -142.8025) -> (171.7475, -142.8025)
  line L379 (171.7475, -142.8025) -> (171.7475, -128.7975)
  line L380 (171.7475, -128.7975) -> (185.7525, -142.8025) construction
  line L381 (185.7525, -128.7975) -> (171.7475, -142.8025) construction
  line L382 (190.7475, -128.7975) -> (204.7525, -128.7975)
  line L383 (204.7525, -128.7975) -> (204.7525, -142.8025)
  line L384 (204.7525, -142.8025) -> (190.7475, -142.8025)
  line L385 (190.7475, -142.8025) -> (190.7475, -128.7975)
  line L386 (190.7475, -128.7975) -> (204.7525, -142.8025) construction
  line L387 (204.7525, -128.7975) -> (190.7475, -142.8025) construction
  line L388 (209.7475, -128.7975) -> (223.7525, -128.7975)
  line L389 (223.7525, -128.7975) -> (223.7525, -142.8025)
  line L390 (223.7525, -142.8025) -> (209.7475, -142.8025)
  line L391 (209.7475, -142.8025) -> (209.7475, -128.7975)
  line L392 (209.7475, -128.7975) -> (223.7525, -142.8025) construction
  line L393 (223.7525, -128.7975) -> (209.7475, -142.8025) construction
  line L394 (228.7475, -128.7975) -> (242.7525, -128.7975)
  line L395 (242.7525, -128.7975) -> (242.7525, -142.8025)
  line L396 (242.7525, -142.8025) -> (228.7475, -142.8025)
  line L397 (228.7475, -142.8025) -> (228.7475, -128.7975)
  line L398 (228.7475, -128.7975) -> (242.7525, -142.8025) construction
  line L399 (242.7525, -128.7975) -> (228.7475, -142.8025) construction
  line L400 (247.7475, -128.7975) -> (261.7525, -128.7975)
  line L401 (261.7525, -128.7975) -> (261.7525, -142.8025)
  line L402 (261.7525, -142.8025) -> (247.7475, -142.8025)
  line L403 (247.7475, -142.8025) -> (247.7475, -128.7975)
  line L404 (247.7475, -128.7975) -> (261.7525, -142.8025) construction
  line L405 (261.7525, -128.7975) -> (247.7475, -142.8025) construction
  line L406 (55.9975, -147.8975) -> (70.0025, -147.8975)
  line L407 (70.0025, -147.8975) -> (70.0025, -161.9025)
  line L408 (70.0025, -161.9025) -> (55.9975, -161.9025)
  line L409 (55.9975, -161.9025) -> (55.9975, -147.8975)
  line L410 (55.9975, -147.8975) -> (70.0025, -161.9025) construction
  line L411 (70.0025, -147.8975) -> (55.9975, -161.9025) construction
  line L412 (80.4975, -147.8975) -> (94.5025, -147.8975)
  line L413 (94.5025, -147.8975) -> (94.5025, -161.9025)
  line L414 (94.5025, -161.9025) -> (80.4975, -161.9025)
  line L415 (80.4975, -161.9025) -> (80.4975, -147.8975)
  line L416 (80.4975, -147.8975) -> (94.5025, -161.9025) construction
  line L417 (94.5025, -147.8975) -> (80.4975, -161.9025) construction
  line L418 (169.8725, -147.8975) -> (183.8775, -147.8975)
  line L419 (183.8775, -147.8975) -> (183.8775, -161.9025)
  line L420 (183.8775, -161.9025) -> (169.8725, -161.9025)
  line L421 (169.8725, -161.9025) -> (169.8725, -147.8975)
  line L422 (169.8725, -147.8975) -> (183.8775, -161.9025) construction
  line L423 (183.8775, -147.8975) -> (169.8725, -161.9025) construction
  line L424 (259.2475, -147.8975) -> (273.2525, -147.8975)
  line L425 (273.2525, -147.8975) -> (273.2525, -161.9025)
  line L426 (273.2525, -161.9025) -> (259.2475, -161.9025)
  line L427 (259.2475, -161.9025) -> (259.2475, -147.8975)
  line L428 (259.2475, -147.8975) -> (273.2525, -161.9025) construction
  line L429 (273.2525, -147.8975) -> (259.2475, -161.9025) construction
  line L430 (45, -90.0975) -> (47, -90.0975)
  line L431 (47, -90.0975) -> (47, -88.5975)
  line L432 (47, -88.5975) -> (49, -88.5975)
  line L433 (49, -88.5975) -> (49, -90.0975)
  line L434 (49, -90.0975) -> (51, -90.0975)
  line L435 (51, -90.0975) -> (51, -102.5975)
  line L436 (51, -102.5975) -> (45, -102.5975)
  line L437 (45, -102.5975) -> (45, -90.0975)
  line L438 (69, -102.1973) -> (75, -102.1973) construction
  line L439 (69, -87.1973) -> (69, -102.1973) construction
  line L440 (75, -102.1973) -> (75, -89.2452) construction
  line L441 (69, -90.0975) -> (71, -90.0975)
  line L442 (71, -90.0975) -> (71, -88.5975)
  line L443 (71, -88.5975) -> (73, -88.5975)
  line L444 (73, -88.5975) -> (73, -90.0975)
  line L445 (73, -90.0975) -> (75, -90.0975)
  line L446 (75, -90.0975) -> (75, -102.5975)
  line L447 (75, -102.5975) -> (69, -102.5975)
  line L448 (69, -102.5975) -> (69, -90.0975)
  line L449 (107.125, -160.2293) -> (113.125, -160.2293) construction
  line L450 (107.125, -145.2293) -> (107.125, -160.2293) construction
  line L451 (113.125, -160.2293) -> (113.125, -147.6329) construction
  line L452 (107.125, -147.3975) -> (109.125, -147.3975)
  line L453 (109.125, -147.3975) -> (109.125, -145.8975)
  line L454 (109.125, -145.8975) -> (111.125, -145.8975)
  line L455 (111.125, -145.8975) -> (111.125, -147.3975)
  line L456 (111.125, -147.3975) -> (113.125, -147.3975)
  line L457 (113.125, -147.3975) -> (113.125, -159.8975)
  line L458 (113.125, -159.8975) -> (107.125, -159.8975)
  line L459 (107.125, -159.8975) -> (107.125, -147.3975)
  line L460 (240.625, -161.1344) -> (246.625, -161.1344) construction
  line L461 (240.625, -146.1344) -> (240.625, -161.1344) construction
  line L462 (246.625, -161.1344) -> (246.625, -147.6329) construction
  line L463 (240.625, -147.3975) -> (242.625, -147.3975)
  line L464 (242.625, -147.3975) -> (242.625, -145.8975)
  line L465 (242.625, -145.8975) -> (244.625, -145.8975)
  line L466 (244.625, -145.8975) -> (244.625, -147.3975)
  line L467 (244.625, -147.3975) -> (246.625, -147.3975)
  line L468 (246.625, -147.3975) -> (246.625, -159.8975)
  line L469 (246.625, -159.8975) -> (240.625, -159.8975)
  line L470 (240.625, -159.8975) -> (240.625, -147.3975)
  line L471 (203, -68.25) -> (160.25, -68.25)
  line L472 (160.25, -68.25) -> (160.25, -61.75)
  line L473 (160.25, -61.75) -> (203, -61.75)
  line L474 (203, -61.75) -> (203, -68.25)
  point P0 (0, 0)
  dimension "d0" = 0.1
  dimension "d1" = 0.1
  dimension "d2" = 0.1
  dimension "d3" = 0.1
  dimension "d4" = 0.1
  dimension "d5" = 0.1
  dimension "d6" = 0.1
  dimension "d7" = 0.1
  dimension "d8" = 0.1
  dimension "d9" = 0.1
  dimension "d10" = 0.1
  dimension "d11" = 14.005
  dimension "d12" = 14.005
  dimension "d13" = 14.005
  dimension "d14" = 14.005
  dimension "d15" = 14.005
  dimension "d16" = 14.005
  dimension "d17" = 14.005
  dimension "d18" = 14.005
  dimension "d19" = 14.005
  dimension "d20" = 14.005
  dimension "d21" = 14.005
  dimension "d22" = 14.005
  dimension "d23" = 14.005
  dimension "d24" = 14.005
  dimension "d25" = 14.005
  dimension "d26" = 14.005
  dimension "d27" = 14.005
  dimension "d28" = 14.005
  dimension "d29" = 14.005
  dimension "d30" = 14.005
  dimension "d31" = 14.005
  dimension "d32" = 14.005
  dimension "d33" = 14.005
  dimension "d34" = 14.005
  dimension "d35" = 14.005
  dimension "d36" = 14.005
  dimension "d37" = 14.005
  dimension "d38" = 14.005
  dimension "d39" = 14.005
  dimension "d40" = 14.005
  dimension "d41" = 14.005
  dimension "d42" = 14.005
  dimension "d43" = 14.005
  dimension "d44" = 14.005
  dimension "d45" = 14.005
  dimension "d46" = 14.005
  dimension "d47" = 14.005
  dimension "d48" = 14.005
  dimension "d49" = 14.005
  dimension "d50" = 14.005
  dimension "d51" = 14.005
  dimension "d52" = 14.005
  dimension "d53" = 14.005
  dimension "d54" = 14.005
  dimension "d55" = 14.005
  dimension "d56" = 14.005
  dimension "d57" = 14.005
  dimension "d58" = 14.005
  dimension "d59" = 14.005
  dimension "d60" = 14.005
  dimension "d61" = 14.005
  dimension "d62" = 14.005
  dimension "d63" = 14.005
  constraints: 894 end point, 122 midpoint, 120 parallel, 110 perpendicular, 63 horizontal, 50 point on line, 33 collinear, 1 vertical
  measures "d0" distance between parallel lines of L37 L75
  measures "d1" distance between parallel lines of L36 L73
  measures "d2" distance between parallel lines of L34 L71
  measures "d3" distance between parallel lines of L32 L69
  measures "d4" distance between parallel lines of L30 L63
  measures "d5" distance between parallel lines of L28 L65
  measures "d6" distance between parallel lines of L29 L64
  measures "d7" distance between parallel lines of L62 L31
  measures "d8" distance between parallel lines of L33 L70
  measures "d9" distance between parallel lines of L72 L35
  measures "d10" distance between parallel lines of L38 L74
  measures "d11" distance of L77.end L78.end
  measures "d12" distance of L76.end L77.end
  measures "d13" distance of L83.end L84.end
  measures "d14" distance of L82.end L83.end
  measures "d15" distance of L89.end L90.end
  measures "d16" distance of L88.end L89.end
  measures "d17" distance of L95.end L96.end
  measures "d18" distance of L94.end L95.end
  measures "d19" distance of L101.end L102.end
  measures "d20" distance of L100.end L101.end
  measures "d21" distance of L107.end L108.end
  measures "d22" distance of L106.end L107.end
  measures "d23" distance of L113.end L114.end
  measures "d24" distance of L112.end L113.end
  measures "d25" distance of L119.end L120.end
  measures "d26" distance of L118.end L119.end
  measures "d27" distance of L125.end L126.end
  measures "d28" distance of L124.end L125.end
  measures "d29" distance of L131.end L132.end
  measures "d30" distance of L130.end L131.end
  measures "d31" distance of L137.end L138.end
  measures "d32" distance of L136.end L137.end
  measures "d33" distance of L143.end L144.end
  measures "d34" distance of L142.end L143.end
  measures "d35" distance of L149.end L150.end
  measures "d36" distance of L148.end L149.end
  measures "d37" distance of L155.end L156.end
  measures "d38" distance of L154.end L155.end
  measures "d39" distance of L161.end L162.end
  measures "d40" distance of L160.end L161.end
  measures "d41" distance of L167.end L168.end